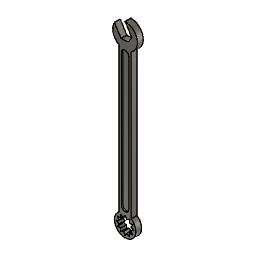
chave combinada v1 (Autodesk Fusion 360 design; units mm, degrees)
Autodesk Fusion 360 part; units mm, degrees
note: some values were not read from the file. Set by a fixed rule: which sketch regions a step uses.
sketch "Sketch1" plane through (0, 0, 0) normal (0, 1, 0) x (1, 0, 0)
  line L0 (0, 0) -> (0, -100)
  circle A0 centre (4.1857, -107.4765) radius 8.5685
  line L1 (4.1857, -1.3614) -> (4.1857, -1.2953)
  line L2 (8.3714, 0) -> (8.3714, -100)
  arc A1 (8.3714, 0) -> (0, 0) centre (4.1857, 6.1156) ccw
  dimension "d1" = 100
  constraint coincident L0.start A1.end
  constraint vertical L0
  constraint coincident L0.end A0
  constraint parallel L0 L1
  measures "d1" distance of L0.start L0.end
extrude "Extrude1" add sketch "Sketch1" along normal blind 5
sketch "Sketch2" plane through (0, 0, 0) normal (0, -1, 0) x (1, 0, 0)
  arc A0 (0, 0) -> (8.3714, 0) centre (4.1857, -6.1156) ccw
  line L0 (8.3714, 0) -> (8.3714, 100)
  arc A1 (8.3714, 100) -> (0, 100) centre (4.1857, 107.4765) ccw
  line L1 (0, 100) -> (0, 0)
  line L2 (3.0876, -2.0175) -> (1.1857, -0.9195)
  line L3 (7.1857, -0.9195) -> (5.2838, -2.0175)
  line L4 (0.0876, -5.0175) -> (-1.8143, -6.1156)
  line L5 (1.1857, -3.1156) -> (-1.0104, -3.1156)
  line L6 (4.1857, -0.1156) -> (3.0876, -2.0175)
  line L7 (0.0876, -7.2137) -> (-1.0104, -9.1156)
  line L8 (1.1857, -0.9195) -> (1.1857, -3.1156)
  line L9 (1.1857, -9.1156) -> (1.1857, -11.3118)
  line L10 (-1.0104, -3.1156) -> (0.0876, -5.0175)
  line L11 (3.0876, -10.2137) -> (4.1857, -12.1156)
  line L12 (-1.8143, -6.1156) -> (0.0876, -7.2137)
  line L13 (5.2838, -10.2137) -> (7.1857, -11.3118)
  line L14 (-1.0104, -9.1156) -> (1.1857, -9.1156)
  line L15 (7.1857, -9.1156) -> (9.3819, -9.1156)
  line L16 (1.1857, -11.3118) -> (3.0876, -10.2137)
  line L17 (8.2838, -7.2137) -> (10.1857, -6.1156)
  line L18 (4.1857, -12.1156) -> (5.2838, -10.2137)
  line L19 (8.2838, -5.0175) -> (9.3819, -3.1156)
  line L20 (7.1857, -11.3118) -> (7.1857, -9.1156)
  line L21 (7.1857, -3.1156) -> (7.1857, -0.9195)
  line L22 (9.3819, -9.1156) -> (8.2838, -7.2137)
  line L23 (5.2838, -2.0175) -> (4.1857, -0.1156)
  line L24 (10.1857, -6.1156) -> (8.2838, -5.0175)
  line L25 (9.3819, -3.1156) -> (7.1857, -3.1156)
  circle A2 centre (4.1857, 107.4765) radius 8.5685
  line L26 (-3.2037, 111.8142) -> (1.4127, 104.4395)
  line L27 (4.1857, 116.045) -> (8.8021, 108.6703)
  spline S0 degree 2 poles (8.8021, 108.6703) (6.4939, 104.4395) (1.4127, 104.4395) knots 0 0 0 0.931949 0.931949 0.931949 weights 1 3 1
  point P0 (4.1857, -6.1156)
  point P1 (4.1857, -6.1156)
  point P2 (4.1857, -6.1156)
  point P3 (4.1857, -6.1156)
  dimension "d5" = 6
  dimension "d6" = 6
  dimension "d7" = 6
  dimension "d8" = 6
  constraint coincident P2 P1
  constraint coincident P3 P2
  constraint collinear L2 L24
  constraint coincident L3.end L22
  constraint collinear L3 L4
  constraint collinear L5 L25
  constraint collinear L6 L7
  constraint collinear L8 L9
  constraint collinear L10 L11
  constraint collinear L12 L13
  constraint collinear L14 L15
  constraint collinear L16 L17
  constraint collinear L18 L19
  constraint collinear L20 L21
  constraint collinear L22 L23
  constraint concentric A1 A2
  constraint coincident A2 L26.start
  constraint coincident A1 L26.start
  constraint midpoint A1 L27.start
  constraint parallel L26 L27
  constraint equal L26 L27
  measures "d5" distance of L6.start P3
  measures "d6" distance of L11.end P3
  measures "d7" distance of L4.end P3
  measures "d8" distance of L17.end P3
extrude "Extrude2" cut sketch "Sketch2" along normal mid plane 18 contours A1 A2 L26 L27 S0 | L2 L3 L4 L5 L6 L7 L8 L9 L10 L11 L12 L13 L14 L15 L16 L17 L18 L19 L20 L21 L22 L23 L24 L25 picked at (4.1836, 108.8223)
sketch "Sketch3" plane through (0, 0, 0) normal (0, -1, 0) x (1, 0, 0)
  line L0 (1.4127, 104.4395) -> (-3.2037, 111.8142)
  arc A0 (-3.2037, 111.8142) -> (0, 100) centre (4.1857, 107.4765) ccw
  line L1 (0, 100) -> (0, 0)
  arc A1 (0, 0) -> (8.3714, 0) centre (4.1857, -6.1156) ccw
  line L2 (8.3714, 0) -> (8.3714, 100)
  arc A2 (8.3714, 100) -> (4.1857, 116.045) centre (4.1857, 107.4765) ccw
  line L3 (4.1857, 116.045) -> (8.8021, 108.6703)
  spline S0 degree 3 poles (8.8021, 108.6703) (7.7372, 106.7184) (7.1677, 105.8398) (6.3827, 105.0938) (6.1105, 104.9214) (5.074, 104.5294) (3.9773, 104.4395) (1.4127, 104.4395) knots 0 0 0 0 0.667054 0.667054 1.004366 1.004366 1.733719 1.733719 1.733719 1.733719
  line L4 (7.1857, -0.9195) -> (7.1857, -3.1156)
  line L5 (7.1857, -3.1156) -> (9.3819, -3.1156)
  line L6 (9.3819, -3.1156) -> (8.2838, -5.0175)
  line L7 (8.2838, -5.0175) -> (10.1857, -6.1156)
  line L8 (10.1857, -6.1156) -> (8.2838, -7.2137)
  line L9 (8.2838, -7.2137) -> (9.3819, -9.1156)
  line L10 (9.3819, -9.1156) -> (7.1857, -9.1156)
  line L11 (7.1857, -9.1156) -> (7.1857, -11.3118)
  line L12 (7.1857, -11.3118) -> (5.2838, -10.2137)
  line L13 (5.2838, -10.2137) -> (4.1857, -12.1156)
  line L14 (4.1857, -12.1156) -> (3.0876, -10.2137)
  line L15 (3.0876, -10.2137) -> (1.1857, -11.3118)
  line L16 (1.1857, -11.3118) -> (1.1857, -9.1156)
  line L17 (1.1857, -9.1156) -> (-1.0104, -9.1156)
  line L18 (-1.0104, -9.1156) -> (0.0876, -7.2137)
  line L19 (0.0876, -7.2137) -> (-1.8143, -6.1156)
  line L20 (-1.8143, -6.1156) -> (0.0876, -5.0175)
  line L21 (0.0876, -5.0175) -> (-1.0104, -3.1156)
  line L22 (-1.0104, -3.1156) -> (1.1857, -3.1156)
  line L23 (1.1857, -3.1156) -> (1.1857, -0.9195)
  line L24 (1.1857, -0.9195) -> (3.0876, -2.0175)
  line L25 (3.0876, -2.0175) -> (4.1857, -0.1156)
  line L26 (4.1857, -0.1156) -> (5.2838, -2.0175)
  line L27 (5.2838, -2.0175) -> (7.1857, -0.9195)
  line L28 (1.6279, 96.2747) -> (1.6245, 4.7564)
  arc A3 (1.6245, 4.7564) -> (6.7471, 4.7562) centre (4.1858, 4.7563) ccw
  line L29 (6.7471, 4.7562) -> (6.7504, 96.2745)
  arc A4 (6.7504, 96.2745) -> (1.6279, 96.2747) centre (4.1891, 96.2746) ccw
  line L30 (4.1892, 98.8359) -> (4.1857, 2.195) construction
  constraint tangent L28 A3
  constraint tangent A3 L29
  constraint parallel L28 L29
  constraint tangent L29 A4
  constraint tangent L28 A4
  constraint midpoint A4 L30.start
  constraint midpoint A3 L30.end
extrude "Extrude3" cut sketch "Sketch3" against normal blind 1 contours L28 A3 L29 A4
extrude "Extrude4" cut 1 faces at (4.1857, 5, 66.6281) along direction (0, -1, 0) blind 1
